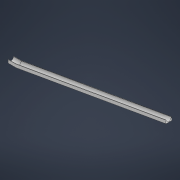
# Autodesk Inventor part: Inverter sentido bolinha
Saved by Autodesk Inventor 2022 (Build 260153000, 153)
## iProperties
Created: 2023-05-08
Part Number: Inverter sentido bolinha
Material: Genérico
Document SubType Name: Modeling
Designer: jpjoa
Density: 1 g/cm^3
Appearance: Padrão
Author: jpjoa
Autodesk Inventor part; units mm, degrees
ref_plane "YZ Plane" through (0, 0, 0) normal (1, 0, 0) x (0, 1, 0)
ref_plane "XZ Plane" through (0, 0, 0) normal (0, 1, 0) x (-1, 0, 0)
ref_plane "XY Plane" through (0, 0, 0) normal (0, 0, 1) x (1, 0, 0)
sketch "Esboço1" plane through (0, 0, 0) normal (0, 0, 1) x (1, 0, 0)
  line L0 (0, 0) -> (9, 0)
  line L1 (9, 0) -> (9, 3.5)
  line L2 (9, 3.5) -> (0, 3.5)
  line L3 (0, 3.5) -> (0, 0)
  line L4 (9, 3.5) -> (9.6171, 0)
  line L5 (9.6171, 0) -> (9, 0)
  line L6 (9.6171, 0) -> (187.8673, 31.4303)
  line L7 (9, 3.5) -> (187.2502, 34.9303)
  line L8 (187.8673, 31.4303) -> (187.2502, 34.9303)
  point P0 (0, 1.75)
  point P1 (4.5, 0)
  dimension "d0" = 3.5
  dimension "d1" = 10
  dimension "d2" = 181
  dimension "d17" = 9
  constraints: 18 end point, 5 perpendicular, 2 horizontal, 2 midpoint, 1 horizontal alignment, 1 parallel, 1 vertical alignment
  measures "d0" distance of L0.end L1.end
  measures "d1" angle of L1 L4
  measures "d2" distance of L4.end L6.end
  measures "d17" distance of L0.start L0.end
extrude "Extrusão1" add sketch "Esboço1" along normal mid plane 7
sketch "Esboço4" plane through (0, 0, 0) normal (0, 0, 1) x (1, 0, 0)
  line L0 (187.2502, 34.9303) -> (9, 3.5) projected
  line L1 (9, 3.5) -> (0, 3.5) projected
  line L2 (187.7711, 31.9759) -> (9.2625, 0.5)
  line L3 (9.2625, 0.5) -> (0, 0.5)
  line L4 (187.7711, 31.9759) -> (187.2502, 34.9303)
  line L5 (0, 0.5) -> (0, 3.5)
  point P0 (0, 0)
  dimension "d13" = 3
  constraints: 8 end point, 1 vertical, 1 other
  measures "d13" distance between parallel lines of L0 L2
extrude "Extrusão4" cut sketch "Esboço4" along normal mid plane 6
fillet "Arredondamento1" radius 3 4 edges at (98.5168, 16.2379, 3) (4.6312, 0.5, 3) (4.6312, 0.5, -3) (98.5168, 16.2379, -3)
